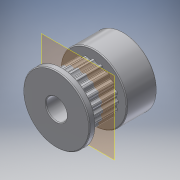
# Autodesk Inventor part: axis plotter motor timing pulley
Saved by Autodesk Inventor 2016 (Build 200138000, 138)
## iProperties
Created: 2017-09-11
Part Number: axis plotter motor timing pulley
Material: ABS Plastic
Document SubType Name: Modeling
Designer: student
Density: 1.06 g/cm^3
Appearance: Smooth - White
Author: student
Autodesk Inventor part; units mm, degrees
ref_plane "YZ Plane" through (0, 0, 0) normal (1, 0, 0) x (0, 1, 0)
ref_plane "XZ Plane" through (0, 0, 0) normal (0, 1, 0) x (-1, 0, 0)
ref_plane "XY Plane" through (0, 0, 0) normal (0, 0, 1) x (1, 0, 0)
sketch "Sketch1" plane through (0, 0, 0) normal (0, 0, 1) x (1, 0, 0)
  circle A0 centre (0, 0) radius 8
  dimension "d0" = 16
  constraints: 1 centre point, 1 coincident
  measures "d0" diameter of A0
extrude "Extrusion1" add sketch "Sketch1" along normal blind 7.25
sketch "Sketch3" plane through (0, 0, 7.25) normal (0, 0, 1) x (1, 0, 0)
  circle A0 centre (0, 0) radius 8
  arc A1 (0.76, 5.5084) -> (-0.76, 5.5084) centre (0, 0) ccw
  arc A2 (0.2634, 5.9737) -> (-0.2634, 5.9737) centre (0, 5.5606) ccw
  arc A3 (-0.76, 5.5084) -> (-0.2634, 5.9737) centre (-1.2509, 6.5301) ccw
  arc A4 (0.2634, 5.9737) -> (0.76, 5.5084) centre (1.2509, 6.5301) ccw
  arc A5 (-2.425, 5.004) -> (-2.0964, 5.5999) centre (-3.2076, 5.824) ccw
  arc A6 (-0.9794, 5.4737) -> (-2.425, 5.004) centre (0, 0) ccw
  arc A7 (-1.5955, 5.7627) -> (-0.9794, 5.4737) centre (-0.8283, 6.5971) ccw
  arc A8 (-1.5955, 5.7627) -> (-2.0964, 5.5999) centre (-1.7183, 5.2884) ccw
  arc A9 (-3.8526, 4.0097) -> (-3.7243, 4.678) centre (-4.8503, 4.5477) ccw
  arc A10 (-2.6229, 4.9031) -> (-3.8526, 4.0097) centre (0, 0) ccw
  arc A11 (-3.2982, 4.9876) -> (-2.6229, 4.9031) centre (-2.8263, 6.0182) ccw
  arc A12 (-3.2982, 4.9876) -> (-3.7243, 4.678) centre (-3.2684, 4.4986) ccw
  arc A13 (-4.9031, 2.6229) -> (-4.9876, 3.2982) centre (-6.0182, 2.8263) ccw
  arc A14 (-4.0097, 3.8526) -> (-4.9031, 2.6229) centre (0, 0) ccw
  arc A15 (-4.678, 3.7243) -> (-4.0097, 3.8526) centre (-4.5477, 4.8503) ccw
  arc A16 (-4.678, 3.7243) -> (-4.9876, 3.2982) centre (-4.4986, 3.2684) ccw
  arc A17 (-5.4737, 0.9794) -> (-5.7627, 1.5955) centre (-6.5971, 0.8283) ccw
  arc A18 (-5.004, 2.425) -> (-5.4737, 0.9794) centre (0, 0) ccw
  arc A19 (-5.5999, 2.0964) -> (-5.004, 2.425) centre (-5.824, 3.2076) ccw
  arc A20 (-5.5999, 2.0964) -> (-5.7627, 1.5955) centre (-5.2884, 1.7183) ccw
  arc A21 (-5.5084, -0.76) -> (-5.9737, -0.2634) centre (-6.5301, -1.2509) ccw
  arc A22 (-5.5084, 0.76) -> (-5.5084, -0.76) centre (0, 0) ccw
  arc A23 (-5.9737, 0.2634) -> (-5.5084, 0.76) centre (-6.5301, 1.2509) ccw
  arc A24 (-5.9737, 0.2634) -> (-5.9737, -0.2634) centre (-5.5606, 0) ccw
  arc A25 (-5.004, -2.425) -> (-5.5999, -2.0964) centre (-5.824, -3.2076) ccw
  arc A26 (-5.4737, -0.9794) -> (-5.004, -2.425) centre (0, 0) ccw
  arc A27 (-5.7627, -1.5955) -> (-5.4737, -0.9794) centre (-6.5971, -0.8283) ccw
  arc A28 (-5.7627, -1.5955) -> (-5.5999, -2.0964) centre (-5.2884, -1.7183) ccw
  arc A29 (-4.0097, -3.8526) -> (-4.678, -3.7243) centre (-4.5477, -4.8503) ccw
  arc A30 (-4.9031, -2.6229) -> (-4.0097, -3.8526) centre (0, 0) ccw
  arc A31 (-4.9876, -3.2982) -> (-4.9031, -2.6229) centre (-6.0182, -2.8263) ccw
  arc A32 (-4.9876, -3.2982) -> (-4.678, -3.7243) centre (-4.4986, -3.2684) ccw
  arc A33 (-2.6229, -4.9031) -> (-3.2982, -4.9876) centre (-2.8263, -6.0182) ccw
  arc A34 (-3.8526, -4.0097) -> (-2.6229, -4.9031) centre (0, 0) ccw
  arc A35 (-3.7243, -4.678) -> (-3.8526, -4.0097) centre (-4.8503, -4.5477) ccw
  arc A36 (-3.7243, -4.678) -> (-3.2982, -4.9876) centre (-3.2684, -4.4986) ccw
  arc A37 (-0.9794, -5.4737) -> (-1.5955, -5.7627) centre (-0.8283, -6.5971) ccw
  arc A38 (-2.425, -5.004) -> (-0.9794, -5.4737) centre (0, 0) ccw
  arc A39 (-2.0964, -5.5999) -> (-2.425, -5.004) centre (-3.2076, -5.824) ccw
  arc A40 (-2.0964, -5.5999) -> (-1.5955, -5.7627) centre (-1.7183, -5.2884) ccw
  arc A41 (0.76, -5.5084) -> (0.2634, -5.9737) centre (1.2509, -6.5301) ccw
  arc A42 (-0.76, -5.5084) -> (0.76, -5.5084) centre (0, 0) ccw
  arc A43 (-0.2634, -5.9737) -> (-0.76, -5.5084) centre (-1.2509, -6.5301) ccw
  arc A44 (-0.2634, -5.9737) -> (0.2634, -5.9737) centre (0, -5.5606) ccw
  arc A45 (2.425, -5.004) -> (2.0964, -5.5999) centre (3.2076, -5.824) ccw
  arc A46 (0.9794, -5.4737) -> (2.425, -5.004) centre (0, 0) ccw
  arc A47 (1.5955, -5.7627) -> (0.9794, -5.4737) centre (0.8283, -6.5971) ccw
  arc A48 (1.5955, -5.7627) -> (2.0964, -5.5999) centre (1.7183, -5.2884) ccw
  arc A49 (3.8526, -4.0097) -> (3.7243, -4.678) centre (4.8503, -4.5477) ccw
  arc A50 (2.6229, -4.9031) -> (3.8526, -4.0097) centre (0, 0) ccw
  arc A51 (3.2982, -4.9876) -> (2.6229, -4.9031) centre (2.8263, -6.0182) ccw
  arc A52 (3.2982, -4.9876) -> (3.7243, -4.678) centre (3.2684, -4.4986) ccw
  arc A53 (4.9031, -2.6229) -> (4.9876, -3.2982) centre (6.0182, -2.8263) ccw
  arc A54 (4.0097, -3.8526) -> (4.9031, -2.6229) centre (0, 0) ccw
  arc A55 (4.678, -3.7243) -> (4.0097, -3.8526) centre (4.5477, -4.8503) ccw
  arc A56 (4.678, -3.7243) -> (4.9876, -3.2982) centre (4.4986, -3.2684) ccw
  arc A57 (5.4737, -0.9794) -> (5.7627, -1.5955) centre (6.5971, -0.8283) ccw
  arc A58 (5.004, -2.425) -> (5.4737, -0.9794) centre (0, 0) ccw
  arc A59 (5.5999, -2.0964) -> (5.004, -2.425) centre (5.824, -3.2076) ccw
  arc A60 (5.5999, -2.0964) -> (5.7627, -1.5955) centre (5.2884, -1.7183) ccw
  arc A61 (5.5084, 0.76) -> (5.9737, 0.2634) centre (6.5301, 1.2509) ccw
  arc A62 (5.5084, -0.76) -> (5.5084, 0.76) centre (0, 0) ccw
  arc A63 (5.9737, -0.2634) -> (5.5084, -0.76) centre (6.5301, -1.2509) ccw
  arc A64 (5.9737, -0.2634) -> (5.9737, 0.2634) centre (5.5606, 0) ccw
  arc A65 (5.004, 2.425) -> (5.5999, 2.0964) centre (5.824, 3.2076) ccw
  arc A66 (5.4737, 0.9794) -> (5.004, 2.425) centre (0, 0) ccw
  arc A67 (5.7627, 1.5955) -> (5.4737, 0.9794) centre (6.5971, 0.8283) ccw
  arc A68 (5.7627, 1.5955) -> (5.5999, 2.0964) centre (5.2884, 1.7183) ccw
  arc A69 (4.0097, 3.8526) -> (4.678, 3.7243) centre (4.5477, 4.8503) ccw
  arc A70 (4.9031, 2.6229) -> (4.0097, 3.8526) centre (0, 0) ccw
  arc A71 (4.9876, 3.2982) -> (4.9031, 2.6229) centre (6.0182, 2.8263) ccw
  arc A72 (4.9876, 3.2982) -> (4.678, 3.7243) centre (4.4986, 3.2684) ccw
  arc A73 (2.6229, 4.9031) -> (3.2982, 4.9876) centre (2.8263, 6.0182) ccw
  arc A74 (3.8526, 4.0097) -> (2.6229, 4.9031) centre (0, 0) ccw
  arc A75 (3.7243, 4.678) -> (3.8526, 4.0097) centre (4.8503, 4.5477) ccw
  arc A76 (3.7243, 4.678) -> (3.2982, 4.9876) centre (3.2684, 4.4986) ccw
  arc A77 (0.9794, 5.4737) -> (1.5955, 5.7627) centre (0.8283, 6.5971) ccw
  arc A78 (2.425, 5.004) -> (0.9794, 5.4737) centre (0, 0) ccw
  arc A79 (2.0964, 5.5999) -> (2.425, 5.004) centre (3.2076, 5.824) ccw
  arc A80 (2.0964, 5.5999) -> (1.5955, 5.7627) centre (1.7183, 5.2884) ccw
  point P0 (0, 6.0505)
  point P1 (-1.8697, 5.7544)
  point P2 (-3.5564, 4.895)
  point P3 (-4.895, 3.5564)
  point P4 (-5.7544, 1.8697)
  point P5 (-6.0505, 0)
  point P6 (-5.7544, -1.8697)
  point P7 (-4.895, -3.5564)
  point P8 (-3.5564, -4.895)
  point P9 (-1.8697, -5.7544)
  point P10 (0, -6.0505)
  point P11 (1.8697, -5.7544)
  point P12 (3.5564, -4.895)
  point P13 (4.895, -3.5564)
  point P14 (5.7544, -1.8697)
  point P15 (6.0505, 0)
  point P16 (5.7544, 1.8697)
  point P17 (4.895, 3.5564)
  point P18 (3.5564, 4.895)
  point P19 (1.8697, 5.7544)
  dimension "d15" = 360
  constraints: 200 point on circle, 81 centre point, 1 coincident, 261 other
extrude "Extrusion2" add sketch "Sketch3" along normal blind 7.5 contours A1 A3 A2 A4 | A5 A8 A7 A6 | A9 A12 A11 A10 | A13 A16 A15 A14 | A17 A20 A19 A18 | A21 A24 A23 A22 | A25 A28 A27 A26 | A29 A32 A31 A30 | A33 A36 A35 A34 | A37 A40 A39 A38 | A41 A44 A43 A42 | A45 A48 A47 A46 | A49 A52 A51 A50 | A53 A56 A55 A54 | A57 A60 A59 A58 | A61 A64 A63 A62 | A65 A68 A67 A66 | A69 A72 A71 A70 | A73 A76 A75 A74 | A77 A80 A79 A78
sketch "Sketch4" plane through (0, 0, 7.25) normal (0, 0, 1) x (1, 0, 0)
  circle A0 centre (0, 0) radius 5.5606
  constraints: 1 centre point, 1 coincident
extrude "Extrusion3" add sketch "Sketch4" along normal blind 7.5
sketch "Sketch5" plane through (0, 0, 14.75) normal (0, 0, 1) x (1, 0, 0)
  circle A0 centre (0, 0) radius 8
  constraints: 1 centre point, 1 coincident
extrude "Extrusion4" add sketch "Sketch5" along normal blind 1.5
sketch "Sketch6" plane through (0, 0, 16.25) normal (0, 0, 1) x (1, 0, 0)
  circle A0 centre (0, 0) radius 2.5
  dimension "d23" = 5
  constraints: 1 centre point, 1 coincident
  measures "d23" diameter of A0
extrude "Extrusion5" cut sketch "Sketch6" against normal through all
fillet "Fillet1" radius 0.2 6 edges at (-2.5, 0, 16.25) (-8, 0, 16.25) (-8, 0, 0) (-8, 0, 7.25) (-8, 0, 14.75) (-2.5, 0, 0)
ref_plane "Work Plane1" through (0, 0, 11) normal (0, 0, 1) x (1, 0, 0)
body "Solid1"
